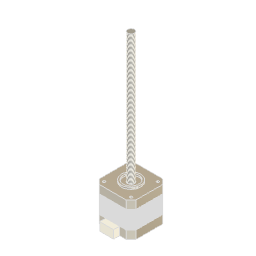
_Clean Plate NEMA 17 w_ Lead Screw.d50ca21d-fa27-44c8-b5f9-0d5c7d1bbd7b (Autodesk Fusion 360 design; units mm, degrees)
Autodesk Fusion 360 part; units mm, degrees
note: some values were not read from the file. Chosen so that the rebuilt part matches the saved one: which bodies a step acts on; how an offset face is resized.
sketch "Sketch1" plane through (0, 0, 0) normal (0, 0, 1) x (1, 0, 0)
  line L0 (21.15, -21.15) -> (-21.15, -21.15)
  line L1 (-21.15, -21.15) -> (-21.15, 21.15)
  line L2 (-21.15, 21.15) -> (21.15, 21.15)
  line L3 (21.15, 21.15) -> (21.15, -21.15)
  line L4 (21.15, -21.15) -> (-21.15, 21.15) construction
  line L5 (-21.15, -21.15) -> (21.15, 21.15) construction
  line L6 (21.15, 15.5) -> (21.15, -15.5)
  line L7 (-21.15, 15.5) -> (-21.15, -15.5)
  line L8 (-15.5, 21.15) -> (15.5, 21.15)
  line L9 (-15.5, -21.15) -> (15.5, -21.15)
  line L10 (15.5, -21.15) -> (21.15, -15.5)
  line L11 (21.15, 15.5) -> (15.5, 21.15)
  line L12 (-21.15, 15.5) -> (-15.5, 21.15)
  line L13 (-21.15, -15.5) -> (-15.5, -21.15)
  dimension "d1" = 42.3
  dimension "d2" = 42.3
  dimension "d4" = 31
  dimension "d5" = 31
  dimension "d6" = 31
  dimension "d7" = 31
  constraint horizontal L0
  constraint perpendicular L0 L1
  constraint parallel L0 L2
  constraint parallel L1 L3
  constraint coincident L4 origin
  constraint coincident L5 origin
  constraint vertical L6
  constraint vertical L7
  constraint perpendicular L1 L8
  constraint midpoint L2 L8
  constraint midpoint L1 L7
  constraint midpoint L3 L6
  constraint horizontal L9
  constraint midpoint L0 L9
  measures "d1" distance of L1.end L2.end
  measures "d2" distance of L0.end L1.end
  measures "d4" distance of L6.end L6.start
  measures "d5" distance of L7.end L7.start
  measures "d6" distance of L8.start L8.end
  measures "d7" distance of L9.start L9.end
extrude "Extrude1" add sketch "Sketch1" along normal blind 39.5 contours L0 L1 L2 L3 L6 L7 L8 L9 L10 L11 L12 L13 makes body 1
ref_plane "WorkPlane1" through (0, 0, 29.9) normal (0, 0, 1) x (1, 0, 0)
ref_plane "WorkPlane2" through (0, 0, 9.6) normal (0, 0, -1) x (-1, 0, 0)
split "Split1" by plane through (0, 0, 29.9) normal (0, 0, 1) and through (0, 0, 9.6) normal (0, 0, -1) bodies 1 makes body 2 at (7.05, -5.1667, 39.5) makes body 3 at (7.05, -5.1667, 0)
sketch "Sketch2" plane through (0, -21.15, 0) normal (0, -1, 0) x (1, 0, 0)
  line L0 (15.5, 9.6) -> (-15.5, 9.6)
  line L1 (-15.5, 9.6) -> (-15.5, 0)
  line L2 (-15.5, 0) -> (15.5, 0)
  line L3 (15.5, 0) -> (15.5, 9.6)
  line L4 (-8, 0) -> (8, 0)
  line L5 (-8, 0) -> (8, 0)
  line L6 (8, 0) -> (8, 9.6)
  line L7 (8, 9.6) -> (-8, 9.6)
  line L8 (-8, 9.6) -> (-8, 0)
  dimension "d12" = 16
  dimension "d13" = 9.6
  constraint horizontal L4
  constraint midpoint L2 L4
  constraint horizontal L5
  constraint vertical L6
  constraint horizontal L7
  constraint vertical L8
  measures "d12" distance of L4.start L4.end
  measures "d13" distance of L4.start L7.end
extrude "Extrude2" add sketch "Sketch2" along normal blind 7 separate body contours L0 L2 L4 L5 L6 L7 L8 makes body 4
ref_plane "WorkPlane3" through (0, 0, 19.75) normal (1, 0, 0) x (0, 1, 0)
sketch "Sketch3" plane through (0, 0, 0) normal (1, 0, 0) x (0, 1, 0)
  line L0 (21.15, 29.9) -> (-21.15, 29.9)
  line L1 (-21.15, 29.9) -> (-21.15, 9.6)
  line L2 (-21.15, 9.6) -> (21.15, 9.6)
  line L3 (21.15, 9.6) -> (21.15, 29.9)
  line L4 (-21.15, 29.9) -> (-20.9, 29.9)
  line L5 (-20.9, 29.9) -> (-20.9, 29.3888)
  line L6 (-20.9, 29.3888) -> (-21.15, 29.3888)
  line L7 (-21.15, 29.3888) -> (-21.15, 29.9)
  dimension "d16" = 0.25
  constraint horizontal L4
  constraint vertical L5
  constraint horizontal L6
  constraint vertical L7
  constraint coincident L0.end L1.start
  measures "d16" distance of L0.end L4.end
sketch "Sketch4" plane through (0, 0, 29.9) normal (0, 0, 1) x (1, 0, 0)
  line L0 (-21.15, 15.5) -> (-21.15, -15.5)
  line L1 (-21.15, -15.5) -> (-15.5, -21.15)
  line L2 (-15.5, -21.15) -> (15.5, -21.15)
  line L3 (15.5, -21.15) -> (21.15, -15.5)
  line L4 (21.15, -15.5) -> (21.15, 15.5)
  line L5 (21.15, 15.5) -> (15.5, 21.15)
  line L6 (15.5, 21.15) -> (-15.5, 21.15)
  line L7 (-15.5, 21.15) -> (-21.15, 15.5)
sweep "Sweep1" cut profiles "Sketch3" path "Sketch4" along L4 L5 L6 L7 L0 L1 L2 L3 section 1 contours L0 L1 L4 L5 L6 L7 bodies 1
pattern_linear "R-Pattern1" count 18 spacing 1.1765 along (0, 0, -1) of "Sweep1"
sketch "Sketch5" plane through (0, 0, 39.5) normal (0, 0, 1) x (-1, 0, 0)
  line L0 (21.15, -15.5) -> (21.15, 15.5)
  line L1 (21.15, 15.5) -> (15.5, 21.15)
  line L2 (15.5, 21.15) -> (-15.5, 21.15)
  line L3 (-15.5, 21.15) -> (-21.15, 15.5)
  line L4 (-21.15, 15.5) -> (-21.15, -15.5)
  line L5 (-21.15, -15.5) -> (-15.5, -21.15)
  line L6 (-15.5, -21.15) -> (15.5, -21.15)
  line L7 (15.5, -21.15) -> (21.15, -15.5)
  circle A0 centre (0, 0) radius 11
  circle A1 centre (0, 0) radius 9
  dimension "d27" = 22
  dimension "d30" = 18
  constraint coincident A0.centre A1.centre
  constraint concentric A0 A1
  measures "d27" diameter of A0
  measures "d30" diameter of A1
extrude "Extrude3" add sketch "Sketch5" along normal blind 2 contours A0 bodies 2
sketch "Sketch6" plane through (0, 0, 39.5) normal (0, 0, 1) x (-1, 0, 0)
  circle A0 centre (0, 0) radius 9
  circle A1 centre (0, 0) radius 4
  dimension "d31" = 8
  constraint concentric A0 A1
  measures "d31" diameter of A1
extrude "Extrude1'" add sketch "Sketch6" along normal blind 150 separate body contours A1 makes body 5 in component "Lead Screw"
copy_body "Body->Comp1" bodies 1 removing the originals makes body 6 in component "NEMA 17"
copy_body "CutPasteBodies1" bodies 2 removing the originals makes body 7 in component "NEMA 17"
copy_body "CutPasteBodies2" bodies 3 removing the originals makes body 8 in component "NEMA 17"
copy_body "CutPasteBodies3" bodies 4 removing the originals makes body 9 in component "NEMA 17"
thread "Thread1" "ISO Metric profile 8.0 M8x1.25 M8x1.25 6g" major diameter 7.866 minor diameter 6.4455 pitch 1.25 angle 60 resizes the face on face at (-3.995, 0.1994, 139.5) on bodies 5 in component "Lead Screw"
sketch "Sketch7" plane through (0, 0, 39.5) normal (0, 0, 1) x (-1, 0, 0)
  line L0 (21.15, -15.5) -> (21.15, 15.5)
  line L1 (21.15, 15.5) -> (15.5, 21.15)
  line L2 (15.5, 21.15) -> (-15.5, 21.15)
  line L3 (-15.5, 21.15) -> (-21.15, 15.5)
  line L4 (-21.15, 15.5) -> (-21.15, -15.5)
  line L5 (-21.15, -15.5) -> (-15.5, -21.15)
  line L6 (-15.5, -21.15) -> (15.5, -21.15)
  line L7 (15.5, -21.15) -> (21.15, -15.5)
  circle A0 centre (0, 0) radius 11
  circle A1 centre (15.5, -15.5) radius 1.4
  circle A2 centre (-15.5, -15.5) radius 1.4
  line L8 (-21.15, 0) -> (21.15, 0) construction
  circle A3 centre (15.5, 15.5) radius 1.4
  circle A4 centre (-15.5, 15.5) radius 1.4
  dimension "d36" = 2.8
  dimension "d37" = 2.8
  constraint midpoint L4 L8.start
  constraint midpoint L0 L8.end
  constraint symmetric A1 L8 A3
  constraint symmetric A2 L8 A4
  measures "d36" diameter of A1
  measures "d37" diameter of A2
extrude "Extrude1''" cut sketch "Sketch7" against normal blind 3 contours A1 | A2 | A3 | A4 bodies 7 in component "NEMA 17"
component "Lead Screw" placed x (1, 0, 0) y (0, 1, 0) z (0, 0, 1) at (0, 0, 0)
component "NEMA 17" placed x (1, 0, 0) y (0, 1, 0) z (0, 0, 1) at (0, 0, 0)
